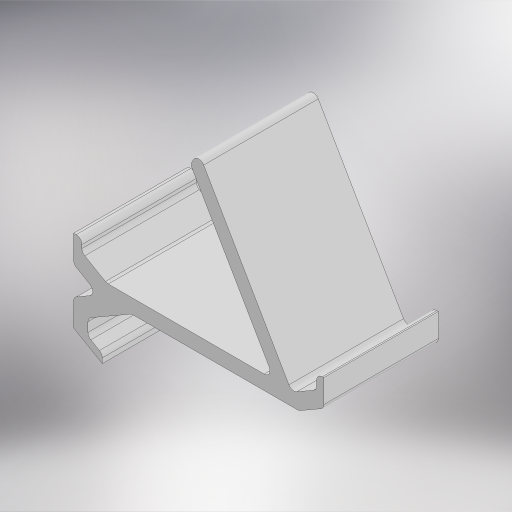
# Autodesk Inventor part: part1
Saved by Autodesk Inventor 2024 (Build 280153000, 153)
## iProperties
Created: 2023-11-13
Part Number: part1
Material: 일반
Document SubType Name: Modeling
Designer: SSAFY
Density: 1 g/cm^3
Appearance: 기본값
Author: SSAFY
Autodesk Inventor part; units mm, degrees
ref_plane "YZ Plane" through (0, 0, 0) normal (1, 0, 0) x (0, 1, 0)
ref_plane "XZ Plane" through (0, 0, 0) normal (0, 1, 0) x (-1, 0, 0)
ref_plane "XY Plane" through (0, 0, 0) normal (0, 0, 1) x (1, 0, 0)
sketch "스케치1" plane through (0, 0, 0) normal (0, 0, 1) x (1, 0, 0)
  line L0 (0, 0) -> (-35, 60.6218)
  line L1 (-35, 60.6218) -> (-70, 0)
  line L2 (-70, 0) -> (0, 0)
  line L3 (-61.3397, 5) -> (-35, 50.6218)
  line L4 (-37.8868, 55.6218) -> (-8.6603, 5)
  line L5 (-8.6603, 5) -> (-67.1132, 5)
  line L6 (0, 0) -> (8.6603, 5)
  line L7 (-2.5, 4.3301) -> (6.1603, 9.3301)
  line L8 (6.1603, 9.3301) -> (8.6603, 5)
  line L9 (6.1603, 9.3301) -> (6.1603, 14.3301)
  line L10 (6.1603, 14.3301) -> (8.6603, 14.3301)
  line L11 (8.6603, 5) -> (8.6603, 14.3301)
  line L12 (-35, 60.6218) -> (-35, 0) construction
  line L13 (-70, 0) -> (-78.6603, 5)
  line L14 (-75.7735, 10) -> (-78.6603, 5)
  line L15 (-75.7735, 14.3301) -> (-78.6603, 14.3301)
  line L16 (-78.6603, 5) -> (-78.6603, 14.3301)
  line L17 (-67.1132, 5) -> (-75.7735, 10)
  line L18 (-75.7735, 10) -> (-75.7735, 14.3301)
  line L19 (-70, 0) -> (-78.6603, -5)
  line L20 (-75.7735, -10) -> (-78.6603, -5)
  line L21 (-78.6603, -5) -> (-78.6603, -14.3301)
  line L22 (-73.6603, -14.3301) -> (-78.6603, -14.3301)
  line L23 (-58.453, 0) -> (-75.7735, -10)
  line L24 (-73.6603, -8.7799) -> (-73.6603, -14.3301)
  line L25 (-73.6603, -14.3301) -> (-68.6603, -17.2169)
  line L26 (-68.6603, -17.2169) -> (-68.6603, -20.1036)
  line L27 (-78.6603, -14.3301) -> (-68.6603, -20.1036)
  point P0 (-76.1603, 9.3301)
  point P1 (-76.1603, 14.3301)
  point P2 (-67.1132, -5)
  point P3 (-76.1603, -9.3301)
  point P4 (-76.1603, -14.3301)
  point P5 (-75.7735, -14.3301)
  dimension "d0" = 60
  dimension "d1" = 60
  dimension "d2" = 70
  dimension "d3" = 5
  dimension "d6" = 90
  dimension "d7" = 5
  dimension "d8" = 10
  dimension "d9" = 5
  dimension "d11" = 5
  dimension "d12" = 120
  dimension "d13" = 5
  constraints: 56 end point, 11 symmetric about line, 10 point on line, 4 perpendicular, 3 midpoint, 3 vertical, 2 parallel, 1 horizontal
  measures "d0" angle of L2 L0
  measures "d1" angle of L2 L1
  measures "d2" distance of L1.end L0.start
  measures "d3" distance between parallel lines of L3 L1
  measures "d6" angle of L6 L0
  measures "d7" distance between parallel lines of L6 L7
  measures "d8" distance between parallel lines of L8 L0
  measures "d9" distance from line of L10 L7.end
  measures "d11" distance between parallel lines of L21 L24
  measures "d12" angle of L25 L24
  measures "d13" distance from line of L25.end L24
extrude "돌출1" add sketch "스케치1" along normal mid plane 40 contours L2 L1 L5 L4 L0 | L0 L7 L8 L6 | L23 L20 L19 L2 | L8 L9 L10 L11 | L13 L14 L17 L1 | L24 L22 L21 L20 L23 | L16 L15 L18 L14 | L25 L26 L27 L22
fillet "모깎기1" radius 2 18 edges at (-75.7735, 10, 0) (-67.1132, 5, 0) (-2.5, 4.3301, 0) (-8.6603, 5, 0) (6.1603, 9.3301, 0) (-37.8868, 55.6218, 0) (-35, 60.6218, 0) (-75.7735, 14.3301, 0) (6.1603, 14.3301, 0) (-78.6603, 5, 0) (-70, 0, 0) (0, 0, 0) (8.6603, 5, 0) (-78.6603, -5, 0) (-58.453, 0, 0) (-73.6603, -8.7799, 0) (-73.6603, -14.3301, 0) (-68.6603, -17.2169, 0)
